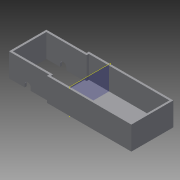
# Autodesk Inventor part: CarChassis
Saved by Autodesk Inventor 2015 (Build 190159000, 159)
## iProperties
Created: 2016-03-26
Part Number: CarChassis
Material: Generic
Document SubType Name: Modeling
Designer: Lee
Density: 1 g/cm^3
Appearance: Default
Author: Lee
Autodesk Inventor part; units mm, degrees
ref_plane "YZ Plane" through (0, 0, 0) normal (1, 0, 0) x (0, 1, 0)
ref_plane "XZ Plane" through (0, 0, 0) normal (0, 1, 0) x (-1, 0, 0)
ref_plane "XY Plane" through (0, 0, 0) normal (0, 0, 1) x (1, 0, 0)
sketch "Sketch1" plane through (0, 0, 0) normal (0, 0, 1) x (1, 0, 0)
  line L0 (0.8, -15.24) -> (-0.8, -15.24)
  line L1 (-0.8, -15.24) -> (-0.8, 15.24)
  line L2 (-0.8, 15.24) -> (0.8, 15.24)
  line L3 (0.8, 15.24) -> (0.8, -15.24)
  line L4 (0.8, -15.24) -> (-0.8, 15.24) construction
  line L5 (-0.8, -15.24) -> (0.8, 15.24) construction
  line L6 (-0.8, -15.24) -> (100.8, -15.24)
  line L7 (100.8, -15.24) -> (100.8, -13.64)
  line L8 (100.8, -13.64) -> (-0.8, -13.64)
  line L9 (-0.8, -13.64) -> (-0.8, -15.24)
  line L10 (-0.8, 15.24) -> (100.8, 15.24)
  line L11 (100.8, 15.24) -> (100.8, 13.64)
  line L12 (100.8, 13.64) -> (-0.8, 13.64)
  line L13 (-0.8, 13.64) -> (-0.8, 15.24)
  line L14 (100.8, -15.24) -> (99.2, -15.24)
  line L15 (99.2, -15.24) -> (99.2, 15.24)
  line L16 (99.2, 15.24) -> (100.8, 15.24)
  line L17 (100.8, 15.24) -> (100.8, -15.24)
  point P0 (0, 0)
  dimension "d0" = 1.6
  dimension "d1" = 30.48
  dimension "d2" = 101.6
  dimension "d3" = 1.6
  dimension "d4" = 101.6
  dimension "d5" = 1.6
  dimension "d6" = 1.6
  constraints: 36 end point, 8 parallel, 4 horizontal, 4 perpendicular, 2 midpoint, 1 point on line
  measures "d0" distance of L1.end L2.end
  measures "d1" distance of L0.end L1.end
  measures "d2" distance of L8.end L7.end
  measures "d3" distance of L7.end L6.end
  measures "d4" distance of L11.end L12.end
  measures "d5" distance of L10.end L11.end
  measures "d6" distance of L15.end L16.end
extrude "Extrusion1" add sketch "Sketch1" along normal blind 19.05 contours L0 L1 L8 L3 | L3 L8 L15 L6 | L8 L1 L12 L3 | L15 L8 L7 L6 | L12 L1 L2 L3 | L3 L10 L15 L12 | L15 L12 L17 L8 | L15 L10 L11 L12
sketch "Sketch2" plane through (-0.8, -15.24, 0) normal (0, -1, 0) x (1, 0, 0)
  line L0 (100, 0) -> (1.6, 0) projected
  line L1 (0, 0) -> (0, 19.05) projected
  line L2 (12.78, 0) -> (17.78, 0)
  line L3 (17.78, 0) -> (17.78, 2.4)
  line L4 (17.78, 2.4) -> (12.78, 2.4)
  line L5 (12.78, 2.4) -> (12.78, 0)
  arc A0 (17.78, 2.4) -> (12.78, 2.4) centre (15.28, 2.4) ccw
  point P0 (0.8, 0)
  dimension "d9" = 12.78
  dimension "d10" = 5
  dimension "d11" = 2.4
  constraints: 8 end point, 2 parallel, 2 point on circle, 2 tangent, 1 centre point, 1 horizontal, 1 perpendicular, 1 point on line
  measures "d9" distance from line of L1 L2.start
  measures "d10" distance of L4.end L3.end
  measures "d11" distance of L3.end L2.end
extrude "Extrusion2" cut sketch "Sketch2" against normal up to surface (30.48 mm away)
ref_plane "Work Plane1" through (50, -15.24, 0) normal (-1, 0, 0) x (0, 0, 1)
sketch "Sketch4" plane through (-0.8, 15.24, 19.05) normal (0, 1, 0) x (1, 0, 0)
  line L0 (12.78, 19.05) -> (17.78, 19.05) projected
  line L1 (17.78, 19.05) -> (12.78, 19.05) projected
  line L2 (48.3, 19.05) -> (32.78, 19.05)
  line L3 (32.78, 19.05) -> (32.78, 18.25)
  line L4 (32.78, 18.25) -> (48.3, 18.25)
  line L5 (48.3, 18.25) -> (48.3, 19.05)
  line L6 (17.78, 19.05) -> (17.78, 16.65) projected
  line L7 (17.78, 19.05) -> (78.82, 19.05)
  line L8 (63.82, 19.05) -> (63.82, 18.25)
  line L9 (63.82, 18.25) -> (48.3, 18.25)
  line L10 (63.82, 19.05) -> (32.78, 19.05)
  line L11 (32.78, 19.05) -> (32.78, 18.25)
  line L12 (32.78, 18.25) -> (63.82, 18.25)
  line L13 (63.82, 18.25) -> (63.82, 19.05)
  point P0 (0.8, 19.05)
  dimension "d15" = 0.8
  dimension "d16" = 15
  constraints: 22 end point, 4 parallel, 4 symmetric about line, 2 horizontal, 2 perpendicular, 1 point on line
  measures "d15" distance of L3.end L2.end
  measures "d16" distance between parallel lines of L6 L3
extrude "Extrusion3" add sketch "Sketch4" against normal up to surface (30.48 mm away)
sketch "Sketch5" plane through (0, 0, 0) normal (0, 0, -1) x (-1, 0, 0)
  line L0 (-99.2, -13.64) -> (-63.02, -13.64) projected
  line L1 (-99.2, 13.64) -> (-99.2, -13.64) projected
  line L2 (-63.02, 13.64) -> (-99.2, 13.64) projected
  line L3 (-63.02, 13.64) -> (-63.02, -13.64) projected
  line L4 (-31.98, 13.64) -> (-31.98, -13.64) projected
  line L5 (-16.98, 13.64) -> (-31.98, 13.64) projected
  line L6 (-16.98, 13.64) -> (-16.98, 15.24) projected
  line L7 (-100.8, 15.24) -> (-16.98, 15.24) projected
  line L8 (-100.8, -15.24) -> (-100.8, 15.24) projected
  line L9 (-16.98, -15.24) -> (-100.8, -15.24) projected
  line L10 (-16.98, -15.24) -> (-16.98, -13.64) projected
  line L11 (-31.98, -13.64) -> (-16.98, -13.64) projected
  line L12 (-11.98, -13.64) -> (-11.98, -15.24) projected
  line L13 (0.8, -15.24) -> (-11.98, -15.24) projected
  line L14 (0.8, 15.24) -> (0.8, -15.24) projected
  line L15 (-11.98, 15.24) -> (0.8, 15.24) projected
  line L16 (-11.98, 15.24) -> (-11.98, 13.64) projected
  line L17 (-0.8, 13.64) -> (-11.98, 13.64) projected
  line L18 (-0.8, -13.64) -> (-0.8, 13.64) projected
  line L19 (-11.98, -13.64) -> (-0.8, -13.64) projected
  line L20 (-100.8, -15.24) -> (-31.966, -15.24)
  line L21 (-31.966, -15.24) -> (-31.966, -17.094)
  line L22 (-31.966, -17.094) -> (-100.8, -17.094)
  line L23 (-100.8, -17.094) -> (-100.8, -15.24)
  point P0 (0, 0)
  dimension "d19" = 32.766
  dimension "d20" = 17.094
  constraints: 8 end point, 2 parallel, 1 horizontal, 1 perpendicular
  measures "d19" distance between parallel lines of L14 L21
  measures "d20" distance from line of L22 point (0, 0)
extrude "Extrusion4" add sketch "Sketch5" against normal up to surface (19.05 mm away) contours L21 L22 L23 L9
sketch "Sketch6" plane through (0, 0, 19.05) normal (0, 0, 1) x (1, 0, 0)
  line L0 (100.8, 15.24) -> (100.8, -17.094) projected
  line L1 (100.8, 15.24) -> (-0.8, 15.24) projected
  line L2 (-0.8, 15.24) -> (-0.8, -15.24) projected
  line L3 (-0.8, -15.24) -> (31.966, -15.24) projected
  line L4 (31.966, -17.094) -> (31.966, -15.24) projected
  line L5 (100.8, -17.094) -> (31.966, -17.094) projected
  line L6 (99.2, 13.64) -> (99.2, -13.64) projected
  line L7 (99.2, -13.64) -> (0.8, -13.64) projected
  line L8 (0.8, -13.64) -> (0.8, 13.64) projected
  line L9 (0.8, 13.64) -> (99.2, 13.64) projected
  line L10 (99.2, -13.64) -> (33.566, -13.64)
  line L11 (33.566, -13.64) -> (33.566, -15.494)
  line L12 (33.566, -15.494) -> (99.2, -15.494)
  line L13 (99.2, -15.494) -> (99.2, -13.64)
  point P0 (0, 0)
  dimension "d23" = 1.6
  dimension "d24" = 1.6
  constraints: 8 end point, 2 parallel, 1 horizontal, 1 perpendicular
  measures "d23" distance between parallel lines of L5 L12
  measures "d24" distance between parallel lines of L11 L4
extrude "Extrusion5" cut sketch "Sketch6" against normal up to surface (18.25 mm away) contours L13 L12 L11 L7
mirror "Mirror3" about plane through (0, 0, 0) normal (0, 1, 0) of "Extrusion4", "Extrusion5"
sketch "Sketch7" plane through (63.02, -13.64, 0) normal (1, 0, 0) x (0, 0, -1)
  line L0 (0, 0) -> (-0.8, 0) projected
  line L1 (0, 27.28) -> (0, 0) projected
  line L2 (-0.8, 27.28) -> (0, 27.28) projected
  line L3 (-0.8, 27.28) -> (-0.8, 0) projected
  point P0 (0, 13.64)
extrude "Extrusion6" add sketch "Sketch7" along normal up to next
body "Solid1"
